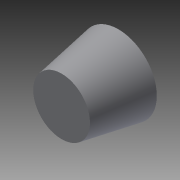
# Autodesk Inventor part: mortar2
Saved by Autodesk Inventor 2015 (Build 190159000, 159)
## iProperties
Created: 2014-07-11
Part Number: mortar2
Material: Generic
Document SubType Name: Modeling
Designer: shohei
Density: 1 g/cm^3
Appearance: Default
Mass: 16749.2 g
Surface Area: 10208.1 cm^2
Volume: 16749.2 cm^3
Author: shohei
Autodesk Inventor part; units mm, degrees
ref_plane "YZ Plane" through (0, 0, 0) normal (1, 0, 0) x (0, 1, 0)
ref_plane "XZ Plane" through (0, 0, 0) normal (0, 1, 0) x (-1, 0, 0)
ref_plane "XY Plane" through (0, 0, 0) normal (0, 0, 1) x (1, 0, 0)
sketch "Sketch1" plane through (0, 0, 0) normal (0, 1, 0) x (-1, 0, 0)
  circle A0 centre (0, 0) radius 175
  dimension "d0" = 350
  constraints: 1 centre point, 1 coincident
  measures "d0" diameter of A0
extrude "Extrusion1" add sketch "Sketch1" along normal blind 350 draft 10
sketch "Sketch3" plane through (0, 350, 0) normal (0, 1, 0) x (1, 0, 0)
  circle A0 centre (0, 0) radius 201.7144
  circle A1 centre (0, 0) radius 236.7144 projected
  dimension "d3" = 35
  constraints: 1 centre point, 1 coincident
  measures "d3" radial gap between concentric circles of A1 A0
extrude "Extrusion2" cut sketch "Sketch3" against normal blind 315 draft -10 contours A0
body "Solid1"
